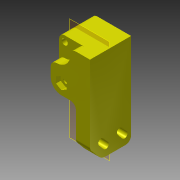
# Autodesk Inventor part: ARM
Saved by Autodesk Inventor 2013 (Build 170138000, 138)
## iProperties
Created: 2013-12-22
Part Number: ARM
Material: Generic
Document SubType Name: Modeling
Designer: employee
Density: 1 g/cm^3
Mass: 7.59464 g
Surface Area: 44.9592 cm^2
Volume: 7.59464 cm^3
Author: employee
Autodesk Inventor part; units mm, degrees
ref_plane "YZ Plane" through (0, 0, 0) normal (1, 0, 0) x (0, 1, 0)
ref_plane "XZ Plane" through (0, 0, 0) normal (0, 1, 0) x (-1, 0, 0)
ref_plane "XY Plane" through (0, 0, 0) normal (0, 0, 1) x (1, 0, 0)
sketch "Sketch1" plane through (0, 0, 0) normal (0, 0, 1) x (1, 0, 0)
  arc A0 (18.8782, 11.9777) -> (7.1013, 4.6885) centre (18.1475, 0) ccw projected
  arc A1 (18.8782, 11.9777) -> (21, 13.974) centre (19, 13.974) ccw projected
  line L0 (21, 13.974) -> (21, 19) projected
  arc A2 (21, 19) -> (19, 21) centre (19, 19) ccw projected
  line L1 (19, 21) -> (-19, 21) projected
  arc A3 (-19, 21) -> (-21, 19) centre (-19, 19) ccw projected
  line L2 (-21, 19) -> (-21, -19) projected
  arc A4 (-21, -19) -> (-19, -21) centre (-19, -19) ccw projected
  line L3 (-19, -21) -> (7.9725, -21) projected
  arc A5 (9.9725, -23) -> (7.9725, -21) centre (7.9725, -23) ccw projected
  line L4 (9.9725, -23.6) -> (9.9725, -23) projected
  arc A6 (9.9725, -23.6) -> (11.9725, -25.6) centre (11.9725, -23.6) ccw projected
  line L5 (19, -25.6) -> (11.9725, -25.6) projected
  arc A7 (19, -25.6) -> (21, -23.6) centre (19, -23.6) ccw projected
  line L6 (21, -13.974) -> (21, -23.6) projected
  arc A8 (21, -13.974) -> (18.8782, -11.9777) centre (19, -13.974) ccw projected
  circle A9 centre (-15.5, 15.5) radius 1.6 projected
  circle A10 centre (15.5, -15.5) radius 1.6 projected
  circle A11 centre (-15.5, -15.5) radius 1.6 projected
  circle A12 centre (15.5, 15.5) radius 1.6 projected
  arc A13 (21, 19) -> (19, 21) centre (19, 19) ccw projected
  line L7 (21, 13.974) -> (21, 19) projected
  arc A14 (18.8782, 11.9777) -> (21, 13.974) centre (19, 13.974) ccw projected
  arc A15 (18.8782, 11.9777) -> (9, 7.7668) centre (18.1475, 0) ccw projected
  line L8 (9, 7.7668) -> (9, 19) projected
  arc A16 (9, 19) -> (7, 21) centre (7, 19) ccw projected
  line L9 (19, 21) -> (7, 21) projected
  circle A17 centre (15.5, 15.5) radius 1.6 projected
  arc A18 (15.5, 18.5) -> (12.5, 15.5) centre (15.5, 15.5) ccw
  arc A19 (12.5, 0) -> (18.1475, -5.6475) centre (18.1475, 0) ccw
  line L10 (12.5, 15.5) -> (12.5, 0)
  line L11 (18.1475, -5.6475) -> (26, -5.6475)
  line L12 (26, -5.6475) -> (26, -31.6)
  line L13 (26, -31.6) -> (33.5, -31.6)
  line L14 (33.5, -31.6) -> (33.5, 18.5)
  line L15 (33.5, 18.5) -> (15.5, 18.5)
  arc A20 (5.4082, 4.4443) -> (7.1013, 4.6885) centre (6.1808, 5.0792) ccw projected
  arc A21 (7.1013, -4.6885) -> (18.8782, -11.9777) centre (18.1475, 0) ccw projected
  arc A22 (7.1013, -4.6885) -> (5.4082, -4.4443) centre (6.1808, -5.0792) ccw projected
  arc A23 (5.4082, 4.4443) -> (5.4082, -4.4443) centre (0, 0) ccw projected
  point P0 (0, 0)
  point P1 (29.75, -31.6)
  dimension "d1" = 7.5
  dimension "d2" = 5
  dimension "d3" = 6
  dimension "d39" = 3
  constraints: 12 end point, 4 perpendicular, 4 point on circle, 4 tangent, 2 centre point, 2 coincident, 1 horizontal alignment, 1 midpoint, 1 parallel
  measures "d1" distance between parallel lines of L14 L12
  measures "d2" distance between parallel lines of L6 L12
  measures "d3" distance between parallel lines of L5 L13
  measures "d39" distance of A12.centre L15.end
extrude "Extrusion1" add sketch "Sketch1" along normal blind 22 contours L10 A18 L15 L0 A1 A0 | A0 A1 L0 L15 L14 L13 L12 L11 A19 L10
sketch "Sketch2" plane through (0, 0, 22) normal (0, 0, 1) x (1, 0, 0)
  circle A0 centre (15.5, 15.5) radius 1.6 projected
  arc A1 (15.5, 18.5) -> (12.5, 15.5) centre (15.5, 15.5) ccw projected
  circle A2 centre (15.5, 15.5) radius 7.5
  point P0 (0, 0)
  dimension "d6" = 15
  constraints: 1 centre point, 1 coincident
  measures "d6" diameter of A2
extrude "Extrusion2" cut sketch "Sketch2" against normal blind 4.5
ref_plane "Work Plane1" through (0, 0, 11) normal (0, 0, 1) x (1, 0, 0)
sketch "Sketch3" plane through (0, 0, 11) normal (0, 0, 1) x (1, 0, 0)
  line L0 (15.5, 18.5) -> (33.5, 18.5) projected
  line L1 (33.5, 18.5) -> (33.5, -31.6) projected
  line L2 (33.5, -31.6) -> (26, -31.6) projected
  line L3 (26, -31.6) -> (26, -5.6475) projected
  line L4 (26, -5.6475) -> (18.1475, -5.6475) projected
  arc A0 (12.5, 0) -> (18.1475, -5.6475) centre (18.1475, 0) ccw projected
  line L5 (12.5, 0) -> (12.5, 15.5) projected
  arc A1 (15.5, 18.5) -> (12.5, 15.5) centre (15.5, 15.5) ccw projected
  circle A2 centre (15.5, 15.5) radius 1.6 projected
  circle A3 centre (18.1475, 0) radius 12.5
  point P0 (0, 0)
  dimension "d11" = 25
  constraints: 1 centre point, 1 coincident
  measures "d11" diameter of A3
extrude "Extrusion3" cut sketch "Sketch3" along normal mid plane 9 contours A3 L3 L4 A0 L5 | L5 A0 L4 L3 A3
sketch "Sketch4" plane through (0, 0, 6.5) normal (0, 0, 1) x (1, 0, 0)
  arc A0 (12.5, 0) -> (18.1475, -5.6475) centre (18.1475, 0) ccw projected
  arc A1 (26, -9.7256) -> (12.5, 11.1515) centre (18.1475, 0) ccw projected
  circle A2 centre (18.1475, 0) radius 5.6475
  point P0 (0, 0)
  constraints: 1 centre point, 1 coincident, 1 concentric
extrude "Extrusion4" add sketch "Sketch4" along normal blind 0.9 draft -45
mirror "Mirror1" about plane through (0, 0, 11) normal (0, 0, 1) of "Extrusion4"
sketch "Sketch5" plane through (0, 0, 22) normal (0, 0, 1) x (1, 0, 0)
  arc A0 (12.5, 0) -> (18.1475, -5.6475) centre (18.1475, 0) ccw projected
  circle A1 centre (18.1475, 0) radius 1.6
  point P0 (0, 0)
  dimension "d18" = 3.2
  constraints: 1 centre point, 1 coincident
  measures "d18" diameter of A1
extrude "Extrusion5" cut sketch "Sketch5" against normal through all
sketch "Sketch6" plane through (0, 0, 0) normal (0, 0, -1) x (-1, 0, 0)
  circle A0 centre (-18.1475, 0) radius 1.6 projected
  arc A1 (-18.1475, -5.6475) -> (-12.5, 0) centre (-18.1475, 0) ccw projected
  circle A2 centre (-18.1475, 0) radius 3
  point P0 (0, 0)
  dimension "d23" = 6
  constraints: 1 centre point, 1 coincident
  measures "d23" diameter of A2
extrude "Extrusion6" cut sketch "Sketch6" against normal blind 3
sketch "Sketch7" plane through (0, 0, 22) normal (0, 0, 1) x (1, 0, 0)
  circle A0 centre (18.1475, 0) radius 1.6 projected
  arc A1 (12.5, 0) -> (18.1475, -5.6475) centre (18.1475, 0) ccw projected
  line L0 (18.1475, 3.262) -> (20.9725, 1.631)
  line L1 (20.9725, 1.631) -> (20.9725, -1.631)
  line L2 (20.9725, -1.631) -> (18.1475, -3.262)
  line L3 (18.1475, -3.262) -> (15.3225, -1.631)
  line L4 (15.3225, -1.631) -> (15.3225, 1.631)
  line L5 (15.3225, 1.631) -> (18.1475, 3.262)
  point P0 (0, 0)
  dimension "d27" = 5.65
  constraints: 12 end point, 1 coincident, 1 vertical, 13 other
  measures "d27" distance between parallel lines of L1 L4
extrude "Extrusion7" cut sketch "Sketch7" against normal blind 2.5
sketch "Sketch8" plane through (33.5, -31.6, 0) normal (1, 0, 0) x (0, 0, -1)
  line L0 (-22, 17.626) -> (0, 17.626) projected
  line L1 (-17.2286, 8) -> (-22, 8) projected
  arc A0 (-14.7539, 10.0285) -> (-17.2286, 8) centre (-15.9796, 9) ccw projected
  line L2 (-14.7539, 10.0285) -> (-13.0518, 8) projected
  line L3 (-7.2286, 8) -> (-13.0518, 8) projected
  arc A1 (-4.7539, 10.0285) -> (-7.2286, 8) centre (-5.9796, 9) ccw projected
  line L4 (-4.7539, 10.0285) -> (-3.0518, 8) projected
  line L5 (0, 8) -> (-3.0518, 8) projected
  line L6 (0, 17.626) -> (0, 8) projected
  line L7 (-13.0518, 8) -> (-12.2843, 7.0853)
  arc A2 (-14.7353, 5.0287) -> (-12.2843, 7.0853) centre (-13.5098, 6.057) ccw
  line L8 (-14.7353, 5.0287) -> (-17.2286, 8)
  line L9 (-3.0518, 8) -> (-2.2607, 7.0571)
  arc A3 (-4.8043, 4.9721) -> (-2.2607, 7.0571) centre (-3.5205, 6) ccw
  line L10 (-4.8043, 4.9721) -> (-7.2286, 8)
  line L11 (-22, 17.626) -> (-22, 8) projected
  point P0 (0, 31.6)
  dimension "d30" = 3
  constraints: 8 end point, 5 tangent, 4 point on circle, 3 parallel, 2 centre point, 1 equal length
  measures "d30" vertical distance of A1.centre A3.centre
extrude "Extrusion8" cut sketch "Sketch8" against normal through all contours A0 L2 L7 A2 L8 | L9 A3 L10 A1 L4
sketch "Sketch9" plane through (33.5, -31.6, 0) normal (1, 0, 0) x (0, 0, -1)
  line L0 (-4.7539, 10.0285) -> (-2.2607, 7.0571) projected
  line L1 (0, 50.1) -> (0, 0) projected
  line L2 (-22, 0) -> (-22, 50.1) projected
  line L3 (0, 0) -> (-22, 0) projected
  line L4 (0, 1.057) -> (-13.5098, 1.057)
  arc A0 (-17.3401, 2.8431) -> (-13.5098, 1.057) centre (-13.5098, 6.057) ccw
  line L5 (-17.3401, 2.8431) -> (-22, 8.3966)
  arc A1 (-14.7353, 5.0287) -> (-12.2843, 7.0853) centre (-13.5098, 6.057) ccw projected
  point P0 (0, 31.6)
  dimension "d33" = 5
  constraints: 4 end point, 2 parallel, 2 point on circle, 2 point on line, 2 tangent, 1 centre point, 1 coincident
  measures "d33" distance from line of A0.centre L4
extrude "Extrusion9" cut sketch "Sketch9" against normal through all
fillet "Fillet1" radius 3 8 edges at (26, -5.6475, 18.75) (26, -5.6475, 3.25) (12.5, 11.1515, 11) (26, -9.7256, 11) (29.75, -23.2034, 22) (29.75, -30.543, 0) (12.5, 8.6261, 19.75) (22.3739, 18.5, 19.75)
body "Solid1"
